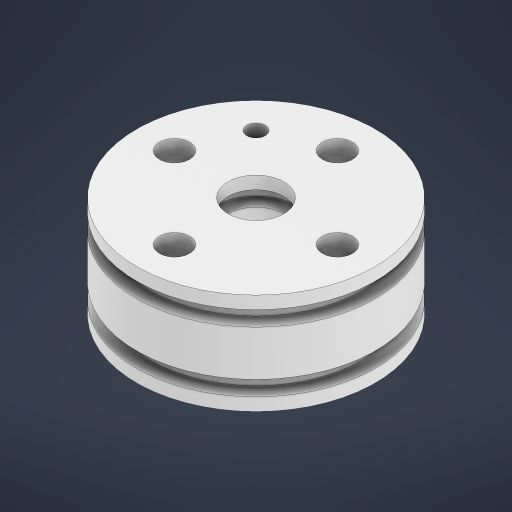
# Autodesk Inventor part: ReserviorPiston
Saved by Autodesk Inventor 2024 (Build 280153000, 153)
## iProperties
Created: 2025-02-07
Part Number: ReserviorPiston
Material: PVC-Piping
Document SubType Name: Modeling
Designer: Tommy Rohmann
Density: 1.4 g/cm^3
Appearance: Smooth - White
Author: Tommy Rohmann
Autodesk Inventor part; units mm, degrees
ref_plane "YZ Plane" through (0, 0, 0) normal (1, 0, 0) x (0, 1, 0)
ref_plane "XZ Plane" through (0, 0, 0) normal (0, 1, 0) x (-1, 0, 0)
ref_plane "XY Plane" through (0, 0, 0) normal (0, 0, 1) x (1, 0, 0)
sketch "ReserviorPiston" plane through (0, 0, 0) normal (0, 0, 1) x (1, 0, 0)
  line L0 (53.5946, 15.2572) -> (53.5946, 20.5912)
  line L1 (53.5946, 20.5912) -> (47.8796, 20.5912)
  line L2 (47.8796, 20.5912) -> (47.8796, 26.9412)
  line L3 (47.8796, 26.9412) -> (53.5946, 26.9412)
  line L4 (53.5946, 26.9412) -> (53.5946, 45.9912)
  line L5 (53.5946, 45.9912) -> (47.8796, 45.9912)
  line L6 (47.8796, 45.9912) -> (47.8796, 52.3412)
  line L7 (47.8796, 52.3412) -> (53.5946, 52.3412)
  line L8 (53.5946, 52.3412) -> (53.5946, 57.6752)
  line L9 (54.2296, 12.8985) -> (54.2296, 63.1281)
  line L10 (3.4296, 2.2226) -> (3.4296, 64.1408)
  line L11 (15.1771, 52.3412) -> (15.1771, 57.6752)
  line L12 (14.5421, 2.6432) -> (14.5421, 52.8728)
  line L13 (20.8921, 45.9912) -> (20.8921, 52.3412)
  line L14 (15.1771, 45.9912) -> (20.8921, 45.9912)
  line L15 (20.8921, 52.3412) -> (15.1771, 52.3412)
  line L16 (15.1771, 26.9412) -> (15.1771, 45.9912)
  line L17 (20.8921, 26.9412) -> (15.1771, 26.9412)
  line L18 (15.1771, 20.5912) -> (20.8921, 20.5912)
  line L19 (20.8921, 20.5912) -> (20.8921, 26.9412)
  line L20 (15.1771, 15.2572) -> (15.1771, 20.5912)
  line L21 (53.5946, 57.6752) -> (15.1771, 57.6752)
  line L22 (53.5946, 15.2572) -> (15.1771, 15.2572)
  line L23 (37.7196, 57.6752) -> (37.7196, 14.7526)
  line L24 (37.7196, 26.9412) -> (44.0696, 26.9412)
  line L25 (44.0696, 26.9412) -> (44.0696, 57.6752)
  line L26 (37.7196, 26.9412) -> (31.3696, 26.9412)
  line L27 (31.3696, 26.9412) -> (31.3696, 57.6752)
  point P0 (34.2963, 101.758)
  dimension "d110" = 0.635
  dimension "d111" = 6.35
  dimension "d112" = 6.35
  dimension "d113" = 19.05
  dimension "d114" = 6.35
  dimension "d118" = 101.6
  dimension "d134" = 0.635
  dimension "d135" = 6.35
  dimension "d136" = 5.334
  dimension "d137" = 5.334
  dimension "d138" = 22.225
  dimension "d145" = 12.7
  dimension "ReserviorPistonHeight" = 42.418
  dimension "d447" = 34.29
  measures "d110" distance between parallel lines of L0 L9
  measures "d111" distance between parallel lines of L7 L5
  measures "d112" distance between parallel lines of L9 L6
  measures "d113" distance of L3.end L4.end
  measures "d114" distance of L1.end L2.end
  measures "d118" diameter of L9 L10
  measures "d134" distance between parallel lines of L12 L11
  measures "d135" distance between parallel lines of L13 L12
  measures "d136" distance between parallel lines of L21 L7
  measures "d137" distance of L0.start L0.end
  measures "d138" diameter of L12 L10
  measures "d145" diameter of L25 L23
  measures "d447" distance between parallel lines of L10 L23
derived "LAYOUT.ipt"
sketch "Sketch1" plane through (0, 0, 0) normal (0, 0, 1) x (1, 0, 0)
  line L0 (53.5946, 15.2572) -> (53.5946, 20.5912)
  line L1 (53.5946, 20.5912) -> (47.8796, 20.5912)
  line L2 (47.8796, 20.5912) -> (47.8796, 26.9412)
  line L3 (47.8796, 26.9412) -> (53.5946, 26.9412)
  line L4 (53.5946, 26.9412) -> (53.5946, 45.9912)
  line L5 (53.5946, 45.9912) -> (47.8796, 45.9912)
  line L6 (47.8796, 45.9912) -> (47.8796, 52.3412)
  line L7 (47.8796, 52.3412) -> (53.5946, 52.3412)
  line L8 (53.5946, 52.3412) -> (53.5946, 57.6752)
  line L9 (54.2296, 12.8985) -> (54.2296, 63.1281)
  line L10 (3.4296, 2.2226) -> (3.4296, 64.1408)
  line L11 (15.1771, 52.3412) -> (15.1771, 57.6752)
  line L12 (14.5421, 2.6432) -> (14.5421, 52.8728)
  line L13 (20.8921, 45.9912) -> (20.8921, 52.3412)
  line L14 (15.1771, 45.9912) -> (20.8921, 45.9912)
  line L15 (20.8921, 52.3412) -> (15.1771, 52.3412)
  line L16 (15.1771, 26.9412) -> (15.1771, 45.9912)
  line L17 (20.8921, 26.9412) -> (15.1771, 26.9412)
  line L18 (15.1771, 20.5912) -> (20.8921, 20.5912)
  line L19 (20.8921, 20.5912) -> (20.8921, 26.9412)
  line L20 (15.1771, 15.2572) -> (15.1771, 20.5912)
  line L21 (53.5946, 57.6752) -> (15.1771, 57.6752)
  line L22 (53.5946, 15.2572) -> (15.1771, 15.2572)
  line L23 (37.7196, 57.6752) -> (37.7196, 14.7526)
  line L24 (37.7196, 26.9412) -> (44.0696, 26.9412)
  line L25 (44.0696, 26.9412) -> (44.0696, 57.6752)
  line L26 (37.7196, 26.9412) -> (31.3696, 26.9412)
  line L27 (31.3696, 26.9412) -> (31.3696, 57.6752)
  point P0 (37.7196, 15.2572)
revolve "Revolution1" add sketch "Sketch1" angle 90 mid plane about axis through (3.4296, 2.2226, 0) along (0, 1, 0)
revolve "Revolution2" cut sketch "Sketch1" angle 360 about axis through (37.7196, 57.6752, 0) along (0, -1, 0) contours L26 L27 L21 L23
pattern_circular "Circular Pattern1" count 4 over 360 about axis through (3.4296, 36.4662, 0) along (0, 1, 0)
sketch "Sketch3" plane through (3.4296, 57.6752, 0) normal (0, 1, 0) x (0, 0, -1)
  circle A0 centre (34.29, 0) radius 6.35 projected
  circle A1 centre (0, 34.29) radius 6.35 projected
  line L0 (0, 34.29) -> (34.29, 0) construction
  line L1 (17.145, 17.145) -> (48.2314, 48.2314) construction
  circle A2 centre (24.5134, 24.5134) radius 3.8735
  circle A3 centre (24.5134, 24.5134) radius 3.175
  dimension "d6" = 7.747
  dimension "d7" = 6.35
  constraints: 4 end point, 2 centre point, 1 coincident, 1 midpoint, 1 point on line
  measures "d6" diameter of A2
  measures "d7" diameter of A3
extrude "Extrusion1" cut sketch "Sketch3" against normal blind 55.5625 contours A3
extrude "Extrusion2" cut sketch "Sketch3" against normal blind 6.35 contours A2
body "Solid1"
